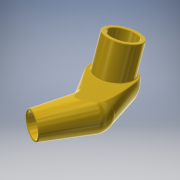
# Autodesk Inventor part: Brazo 1 Lego
Saved by Autodesk Inventor 2017 (Build 210142000, 142)
## iProperties
Created: 2017-06-23
Part Number: Brazo 1 Lego
Material: Plástico ABS
Document SubType Name: Modeling
Designer: H. Valenzuela B.
Density: 1.06 g/cm^3
Appearance: Suave - Blanco
Author: H. Valenzuela B.
Autodesk Inventor part; units mm, degrees
ref_plane "YZ Plane" through (0, 0, 0) normal (1, 0, 0) x (0, 1, 0)
ref_plane "XZ Plane" through (0, 0, 0) normal (0, 1, 0) x (-1, 0, 0)
sketch "Boceto1" plane through (0, 0, 0) normal (0, 0, 1) x (1, 0, 0)
  line L0 (0, 0) -> (2, -4.241888)
  line L1 (2, -4.241888) -> (-0.177994, -9.418262)
  line L2 (-0.177994, -9.418262) -> (1.204606, -10)
  line L3 (1.204606, -10) -> (3.766063, -5.180514)
  arc A0 (1.147073, -2.432878) -> (1.22435, -6.085354) centre (2, -4.241888) ccw construction
  line L4 (2, -4.241888) -> (2.77565, -2.398422)
  arc A1 (2.77565, -2.398422) -> (1.147073, -2.432878) centre (2, -4.241888) ccw construction
  arc A2 (1.22435, -6.085354) -> (2.77565, -2.398422) centre (2, -4.241888) ccw
  line L5 (1.22435, -6.085354) -> (2.77565, -2.398422)
  dimension "d4" = 10
  dimension "d5" = 2
  dimension "d6" = 2
  dimension "d11" = 3
  constraints: 12 end point, 8 point on circle, 3 centre point, 2 coincident, 2 point on line, 2 tangent, 1 collinear, 1 perpendicular
  measures "d4" vertical distance of L2.end point (0, 0)
  measures "d5" radius of A2
  measures "d6" horizontal distance of point (0, 0) L0.end
  measures "d11" diameter of L2.end L1
revolve "Revolución1" add sketch "Boceto1" angle 360 about axis through (2, -4.241888, 0) along (-0.3878252, -0.9217329, 0)
sketch "Boceto2" plane through (0, 0, 0) normal (0, 0, 1) x (1, 0, 0)
  line L0 (2, -4.241888) -> (0, 0)
  line L1 (0, -8.868028) -> (0, 5.359995) construction
  line L2 (-4.499585, 0) -> (6.188857, 0) construction
  arc A0 (3.766063, -5.180514) -> (0.094134, -3.635526) centre (2, -4.241888) ccw
  arc A1 (0, -2.5) -> (1.066158, -2.261262) centre (0, 0) ccw
  line L3 (2.364135, 0.812937) -> (3.80901, -3.388961)
  arc A2 (0, -4.241888) -> (2.852927, -6.050897) centre (2, -4.241888) ccw
  line L4 (2.852927, -6.050897) -> (-1.066158, 2.261262)
  arc A3 (-1.066158, 2.261262) -> (0, -2.5) centre (0, 0) ccw
  arc A4 (1.066158, -2.261262) -> (-1.066158, 2.261262) centre (0, 0) ccw
  arc A5 (1.147073, -2.432878) -> (0, -4.241888) centre (2, -4.241888) ccw
  arc A6 (2.852927, -6.050897) -> (1.147073, -2.432878) centre (2, -4.241888) ccw
  dimension "d8" = 5
  constraints: 17 point on circle, 6 centre point, 6 end point, 5 point on line, 2 coincident, 2 tangent, 1 collinear
  measures "d8" diameter of A1
sketch "Boceto2 outline for Revolución2" plane through (0, 0, 0) normal (0, 0, 1) x (1, 0, 0)
  line L0 (3.80901, -3.388961) -> (2.364135, 0.812937)
  arc A0 (2.364135, 0.812937) -> (-1.066158, 2.261262) centre (0, 0) ccw
  line L1 (-1.066158, 2.261262) -> (2.852927, -6.050897)
  arc A1 (2.852927, -6.050897) -> (3.80901, -3.388961) centre (2, -4.241888) ccw
revolve "Revolución2" add sketch "Boceto2 outline for Revolución2" angle 360 about axis through (2.852927, -6.050897, 0) along (-0.4264634, 0.9045048, 0)
sketch "Boceto3" plane through (0, 0, 0) normal (1, 0, 0) x (0, 1, 0)
  line L0 (4.731079, 0.019998) -> (-7.348692, 2.149987)
  line L1 (-7.348692, 2.149987) -> (-6.61637, 6.303191)
  line L2 (-6.61637, 6.303191) -> (5.4634, 4.173202)
  line L3 (5.4634, 4.173202) -> (4.731079, 0.019998)
  line L4 (-13.05283, 0) -> (8.510215, 0) construction
  line L5 (-13.111468, 0) -> (8.862045, 0) construction
  line L6 (0, 8.02249) -> (0, -4.253748) construction
  point P0 (0, 0)
  dimension "d21" = 10
  constraints: 8 end point, 2 parallel, 1 perpendicular
  measures "d21" angle of L0 L4
extrude "Extrusión1" cut sketch "Boceto3" along normal through all both and the other way through all
sketch "Boceto4" plane through (-0.177994, -9.418262, 0) normal (-0.3878252, -0.9217329, 0) x (0.9217329, -0.3878252, 0)
  circle A0 centre (0, 0) radius 1.5 projected
  circle A1 centre (0, 0) radius 1.275
  point P0 (-3.488577, 0)
  dimension "d12" = 2.55
  constraints: 1 centre point, 1 coincident
  measures "d12" diameter of A1
extrude "Extrusión2" cut sketch "Boceto4" against normal blind 5 contours A1
fillet "Empalme1" radius 1.5 2 edges at (3.6511, -3.4634, -0.8173) (-0.086, -4.4896, -0.5726)
fillet "Empalme2" radius 0.1 6 edges at (2.8885, -1.709, 1.1556) (-0.678, -2.8256, 1.3524) (-1.0166, 2.2372, 0.4597) (0.5867, -4.3133, 0) (-1.5606, -8.8365, 0) (-1.3532, -8.9238, 0)
sketch "Boceto6" plane through (0, 0, 0) normal (1, 0, 0) x (0, 1, 0)
  arc A0 (-0.301725, -2.481726) -> (2.475732, 0.347495) centre (0, 0) ccw
  line L0 (0, 0) -> (1.467706, 4.160405)
  line L1 (2.448747, 1.465821) -> (2.178952, 0.701052)
  line L2 (1.467706, 4.160405) -> (3.344352, 3.498363)
  line L3 (3.344352, 3.498363) -> (1.876646, -0.662042)
  line L4 (1.876646, -0.662042) -> (0, 0)
  line L5 (-1.151236, 1.057209) -> (2.394067, 0.432076)
  point P0 (0.762682, 0.719733)
  dimension "d22" = 3.98
  constraints: 10 end point, 2 perpendicular, 1 parallel, 3 other
  measures "d22" diameter of L3 L0
revolve "Revolución3" add sketch "Boceto6" angle 360 about axis through (0, 0, 0) along (0, 0.3326847, 0.9430381)
sketch "Boceto7" plane through (0, 1.467706, 4.160405) normal (0, 0.3326847, 0.9430381) x (1, 0, 0)
  circle A0 centre (0, 0) radius 1.5
  dimension "d24" = 3
  constraints: 1 centre point, 1 coincident
  measures "d24" diameter of A0
extrude "Extrusión4" cut sketch "Boceto7" against normal blind 3
fillet "Empalme3" radius 0.1 4 edges at (0, -1.7029, 1.1545) (0, -0.4089, 4.8224) (-1.5, 1.4677, 4.1604) (-1.5, 0.469, 1.3294)
ref_plane "Plano de trabajo1" through (0, 1.467706, 4.160405) normal (0, 0.3326847, 0.9430381) x (1, 0, 0)
